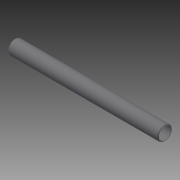
# Autodesk Inventor part: 02-6.3880-nr
Saved by Autodesk Inventor 2013 (Build 170138000, 138)
## iProperties
Created: 2013-01-26
Part Number: 02-6.3880-nr
Material: Generic
Catalog Web Link: www.cadenas.de
Description: NR Tube-Original Line Cylinders
Vendor: BIMBA
Document SubType Name: Modeling
Designer: actoennies
Manufacturer: BIMBA
Density: 1 g/cm^3
Category: PARTsolutions
Company: BIMBA
Title: 02-6.3880-nr
Author: Cadenas PARTsolutions
Comments: Original Line Cylinders
PSOL_IDENT_0: {\\10.0.0.242\data_v9\23d-libs\bimba\bimba\bimba_imperial\bimba_full_line\original_line_cylinders\no
PSOL_IDENT_1: n_rotating_air_cylinders\non_rot_tube.prj},192 {VTYP=3D},{NB=02-6.3880-nr},{LINA=02-6.3880-nr},{NN=N
PSOL_IDENT_2: R Tube},{DATE=20.08.2011 07:16:43},{GEOMDATE=28.02.2011 00:00:00},{VERSION=},{LINEID=30},{LINESUBID=
PSOL_IDENT_3: -1},{WBVAR=MNT,ACTING,L,FOURHOLES,SR}  {NB=02-6.3880-nr},{LINA=02-6.3880-nr},{KT=DUMMY},{PN=02-6.388
PSOL_IDENT_4: 0-nr},{BORE=0.56250000},{BOREPN=02},{MNT=},{MNTALG='' , 'Front Nose'},{ACTING=},{ACTINGALG= '' , 'Si
PSOL_IDENT_5: ngle Acting' , 'R' , 'Reverse/Double Acting' },{NR=},{NRALG= '' , 'Without Non-rotating Rod' , 'NR'
PSOL_IDENT_6: , 'With Non-rotating Rod' },{L=6.3880},{OD=0.6150},{ODN=0.6150},{ODP=0.6150},{ODB=0.0000},{ID=0.5725
PSOL_IDENT_7: },{DV=0.00000000},{LV=0.00000000},{LV1=0.00000000},{G=0.0250},{FOURHOLES=0},{AA=0.3750},{BB=0.0940},
PSOL_IDENT_8: {SR=},{SRALG= 'C' , 'Carbon Steel Rod' , 'SR' , '303 Stainless Steel Rod' , '' , '303 Stainless Stee
PSOL_IDENT_9: l Rod'},{COLOR=0.71,0.71,0.71,0.00}
CNS_NT: Original Line Cylinders
CNS_NB: 02-6.3880-nr
CNS_NBSYN: $PN.
CNS_LINA: 02-6.3880-nr
CNS_PN: 02-6.3880-nr
CNS_BORE: 0.56250000
CNS_BOREPN: 02
CNS_MNT: Front Nose
CNS_MNTALG: '' , 'Front Nose'
CNS_ACTING: Single Acting
CNS_ACTINGALG: '' , 'Single Acting' , 'R' , 'Reverse/Double Acting'
CNS_NRALG: '' , 'Without Non-rotating Rod' , 'NR' , 'With Non-rotating Rod'
CNS_L: 6.3880
CNS_OD: 0.6150
CNS_ODN: 0.6150
CNS_ODP: 0.6150
CNS_ODB: 0.0000
CNS_ID: 0.5725
CNS_DV: 0.00000000
CNS_LV: 0.00000000
CNS_LV1: 0.00000000
CNS_G: 0.0250
CNS_FOURHOLES: 0
CNS_AA: 0.3750
CNS_BB: 0.0940
CNS_SR: 303 Stainless Steel Rod
CNS_SRALG: 'C' , 'Carbon Steel Rod' , 'SR' , '303 Stainless Steel Rod' , '' , '303 Stainless Steel Rod'
CNS_COLOR: 0.71,0.71,0.71,0.00
SUPPLIER: BIMBA
ARTICLENO: 02-6.3880-nr
BOMINFO: 02-6.3880-nr
CREATOR: CADENAS GmbH
Autodesk Inventor part; units mm, degrees
ref_plane "YZ Plane" through (0, 0, 0) normal (1, 0, 0) x (0, 1, 0)
ref_plane "XZ Plane" through (0, 0, 0) normal (0, 1, 0) x (-1, 0, 0)
ref_plane "XY Plane" through (0, 0, 0) normal (0, 0, 1) x (1, 0, 0)
sketch "Sketch_1" plane through (0, 0, 0) normal (0, 0, 1) x (1, 0, 0)
  line L0 (162.2552, 0) -> (0, 0)
  arc A0 (-0.518, 7.0158) -> (-0.518, 6.8362) centre (-0.4282, 6.926) ccw
  line L1 (-0.518, 6.8362) -> (-0.3175, 6.6357)
  line L2 (-0.3175, 6.6357) -> (0, 6.6357)
  line L3 (0, 6.6357) -> (0.635, 7.2708)
  line L4 (0.635, 7.2708) -> (161.6202, 7.2708)
  line L5 (161.6202, 7.2708) -> (162.2552, 6.6357)
  line L6 (162.2552, 6.6357) -> (162.5727, 6.6357)
  line L7 (162.5727, 6.6357) -> (162.7732, 6.8362)
  arc A1 (162.7732, 6.8362) -> (162.7732, 7.0158) centre (162.6834, 6.926) ccw
  line L8 (162.7732, 7.0158) -> (162.1645, 7.6245)
  arc A2 (162.1645, 7.6245) -> (161.7155, 7.8105) centre (161.7154, 7.1755) ccw
  line L9 (161.7155, 7.8105) -> (0.5398, 7.8105)
  arc A3 (0.5398, 7.8105) -> (0.0907, 7.6245) centre (0.5397, 7.1755) ccw
  line L10 (0.0907, 7.6245) -> (-0.518, 7.0158)
  constraints: 22 end point, 8 point on circle, 4 centre point
revolve "Revolution1" add sketch "Sketch_1" angle 360 about axis through (162.2552, 0, 0) along (1, 0, 0)
ref_plane "tube_front_XY" through (0, 0, 0) normal (1, 0, 0) x (0, 0, -1)
ref_plane "tube_front_YZ" through (0, 0, 0) normal (0, 0, -1) x (0, 1, 0)
ref_plane "tube_front_ZX" through (0, 0, 0) normal (0, 1, 0) x (1, 0, 0)
ref_plane "tube_rear_XY" through (162.2552, 0, 0) normal (1, 0, 0) x (0, 0, -1)
ref_plane "tube_rear_YZ" through (162.2552, 0, 0) normal (0, 0, -1) x (0, 1, 0)
ref_plane "tube_rear_ZX" through (162.2552, 0, 0) normal (0, 1, 0) x (1, 0, 0)
ref_plane "cp1_XY" through (81.1276, 7.8105, 0) normal (1, 0, 0) x (0, 0, -1)
ref_plane "cp1_YZ" through (81.1276, 7.8105, 0) normal (0, 0, -1) x (0, 1, 0)
ref_plane "cp1_ZX" through (81.1276, 7.8105, 0) normal (0, 1, 0) x (1, 0, 0)
ref_plane "cp2_XY" through (81.1276, 0, -7.8105) normal (1, 0, 0) x (0, 0, -1)
ref_plane "cp2_YZ" through (81.1276, 0, -7.8105) normal (0, 0, -1) x (0, 1, 0)
ref_plane "cp2_ZX" through (81.1276, 0, -7.8105) normal (0, 1, 0) x (1, 0, 0)
ref_plane "cp3_XY" through (81.1276, -7.8105, 0) normal (1, 0, 0) x (0, 0, -1)
ref_plane "cp3_YZ" through (81.1276, -7.8105, 0) normal (0, 0, -1) x (0, 1, 0)
ref_plane "cp3_ZX" through (81.1276, -7.8105, 0) normal (0, 1, 0) x (1, 0, 0)
ref_plane "cp4_XY" through (81.1276, 0, 7.8105) normal (1, 0, 0) x (0, 0, -1)
ref_plane "cp4_YZ" through (81.1276, 0, 7.8105) normal (0, 0, -1) x (0, 1, 0)
ref_plane "cp4_ZX" through (81.1276, 0, 7.8105) normal (0, 1, 0) x (1, 0, 0)
body "Solid1"
